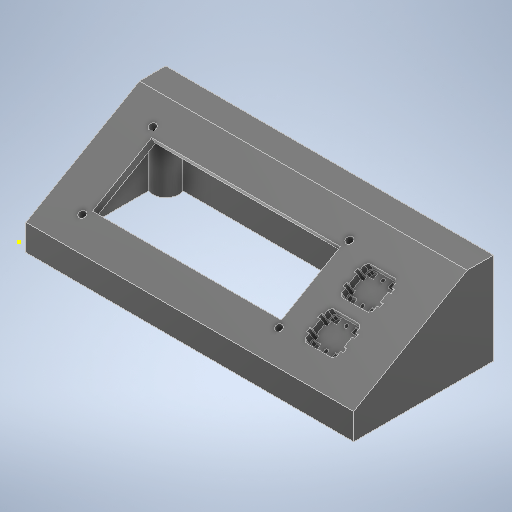
# Autodesk Inventor part: Control_Mount
Saved by Autodesk Inventor 2025.1 (Build 291241020, 241B)
## iProperties
Created: 2024-11-21
Part Number: Control_Mount
Material: PC/ABS Plastic
Document SubType Name: Modeling
Designer: leon-
Density: 1.1 g/cm^3
Appearance: Smooth - Black
Author: leon-
## iProperties of the stored document Control_Mount_3DPrint.ipt
Created: 2024-11-21
Part Number: Control_Mount_3DPrint
Material: Generic
Document SubType Name: Modeling
Designer: leon-
Density: 1 g/cm^3
Appearance: Default
Author: leon-
Autodesk Inventor part; units mm, degrees
ref_plane "YZ Plane" through (0, 0, 0) normal (1, 0, 0) x (0, 1, 0)
ref_plane "XZ Plane" through (0, 0, 0) normal (0, 1, 0) x (-1, 0, 0)
ref_plane "XY Plane" through (0, 0, 0) normal (0, 0, 1) x (1, 0, 0)
sketch "Sketch1" plane through (0, 0, 0) normal (1, 0, 0) x (0, 1, 0)
  line L0 (0, 0) -> (0, -53.3013)
  line L1 (0, -53.3013) -> (35, -53.3013)
  line L2 (35, -53.3013) -> (35, -43.3013)
  line L3 (35, -43.3013) -> (10, 0)
  line L4 (10, 0) -> (0, 0)
  point P0 (5, 0)
  dimension "d0" = 10
  dimension "d2" = 30
  dimension "d3" = 10
  dimension "d7" = 50
  constraints: 10 end point, 2 perpendicular, 1 midpoint, 1 parallel, 1 vertical
  measures "d0" distance of L1.end L2.end
  measures "d2" angle of L0 L3
  measures "d3" distance of L3.end L0.start
  measures "d7" distance of L2.end L3.end
extrude "Extrusion1" add sketch "Sketch1" along normal blind 125
shell "Shell1" thickness 3 removed faces 1 at (41.6667, 0, -17.7671)
sketch "Sketch2" plane through (0, 10, 0) normal (0, 0.8660254, 0.5) x (1, 0, 0)
  line L0 (15, 38) -> (87, 38)
  line L1 (87, 38) -> (87, 12)
  line L2 (87, 12) -> (15, 12)
  line L3 (15, 12) -> (15, 38)
  line L4 (125, 50) -> (125, 0) projected
  line L5 (0, 0) -> (125, 0) projected
  line L6 (0, 50) -> (0, 0) projected
  point P0 (0, -5)
  dimension "d8" = 26
  dimension "d9" = 72
  dimension "d11" = 12
  dimension "d25" = 15
  constraints: 8 end point, 2 parallel, 1 horizontal, 1 perpendicular
  measures "d8" distance of L0.end L1.end
  measures "d9" distance of L0.start L0.end
  measures "d11" distance between parallel lines of L5 L2
  measures "d25" distance between parallel lines of L6 L3
extrude "Extrusion2" cut sketch "Sketch2" against normal up to surface (3 mm away)
ref_plane "Work Plane1" through (87, 22.5, -21.6506) normal (0, 0.5, -0.8660254) x (-1, 0, 0)
ref_plane "Work Plane2" through (51, 16, -10.3923) normal (1, 0, 0) x (0, 0.5, -0.8660254)
sketch "Sketch3" plane through (0, 10, 0) normal (0, 0.8660254, 0.5) x (1, 0, 0)
  line L0 (51, 72.1423) -> (51, -22.2321) projected
  line L1 (-25, 25) -> (150, 25) projected
  point P0 (0, -5)
  point P1 (13, 40.8)
  point P2 (88, 40.8)
  point P3 (88, 9.8)
  point P4 (13, 9.8)
  dimension "d14" = 75
  dimension "d15" = 31
  dimension "d16" = 37
  dimension "d17" = 15.8
  constraints: 2 horizontal alignment, 2 vertical alignment
  measures "d14" distance of point (88, 40.8) point (13, 40.8)
  measures "d15" distance of point (88, 40.8) point (88, 9.8)
  measures "d16" distance from line of point (88, 40.8) L0
  measures "d17" distance from line of L1 point (88, 40.8)
hole "Hole1" at (13, 30.4, -35.3338) at (88, 30.4, -35.3338) at (88, 14.9, -8.487) at (13, 14.9, -8.487) direction (0, -0.8660254, -0.5) diameter 2.6 depth 3
sketch "Sketch4" plane through (3, 32, -44.1051) normal (0, -0.8660254, -0.5) x (1, 0, 0)
  line L0 (110, 7.1962) -> (90, 7.1962)
  line L1 (90, 7.1962) -> (90, 43.1962)
  line L2 (90, 43.1962) -> (110, 43.1962)
  line L3 (110, 43.1962) -> (110, 7.1962)
  line L4 (84, 37.1962) -> (12, 37.1962) projected
  line L5 (84, 11.1962) -> (84, 37.1962) projected
  line L6 (12, 11.1962) -> (84, 11.1962) projected
  point P0 (-3, 54.1962)
  dimension "d76" = 20
  dimension "d78" = 6
  dimension "d79" = 6
  dimension "d80" = 4
  constraints: 8 end point, 2 parallel, 1 horizontal, 1 perpendicular
  measures "d76" distance of L0.start L0.end
  measures "d78" distance between parallel lines of L4 L2
  measures "d79" distance between parallel lines of L5 L1
  measures "d80" distance between parallel lines of L6 L0
extrude "Extrusion3" add sketch "Sketch4" along normal blind 3
sketch "Sketch5" plane through (0, 10, 0) normal (0, 0.8660254, 0.5) x (1, 0, 0)
  line L0 (108, 22) -> (98, 22)
  line L1 (97, 21) -> (98, 22)
  line L2 (97, 21) -> (97, 11)
  line L3 (98, 10) -> (97, 11)
  line L4 (98, 10) -> (108, 10)
  line L5 (109, 11) -> (108, 10)
  line L6 (109, 11) -> (109, 21)
  line L7 (108, 22) -> (109, 21)
  circle A0 centre (103, 16) radius 3.5
  line L8 (87, 38) -> (87, 12) projected
  line L9 (87, 12) -> (15, 12) projected
  point P0 (0, -5)
  point P1 (98, 19.4445)
  point P2 (97, 16)
  dimension "d32" = 12
  dimension "d33" = 12
  dimension "d34" = 7
  dimension "d35" = 6
  dimension "d36" = 6
  dimension "d37" = 1
  dimension "d38" = 1
  dimension "d60" = 10
  dimension "d81" = 2
  constraints: 16 end point, 3 perpendicular, 2 horizontal alignment, 2 vertical alignment, 1 centre point, 1 midpoint
  measures "d32" distance between parallel lines of L6 L2
  measures "d33" distance between parallel lines of L4 L0
  measures "d34" diameter of A0
  measures "d35" distance from line of L6 A0.centre
  measures "d36" distance from line of L0 A0.centre
  measures "d37" horizontal distance of L0.start L6.end
  measures "d38" horizontal distance of L0.start L6.end
  measures "d60" distance from line of L8 point (97, 16)
  measures "d81" distance between parallel lines of L9 L4
ref_plane "Work Plane3" through (98, 19.7222, -16.8394) normal (1, 0, 0) x (0, 0, -1)
ref_plane "Work Plane4" through (92, 18.6328, -20.9325) normal (0, -0.8660254, -0.5) x (1, 0, 0)
extrude "Extrusion4" cut sketch "Sketch5" against normal up to surface (2.99 mm away) contours L7 L6 L5 L4 L3 L2 L1 L0 | A0
sketch "Sketch8" plane through (93, 20.1328, -23.5306) normal (0, 0.8660254, 0.5) x (1, 0, 0)
  line L0 (15.5, -5.9445) -> (12.8, -5.9445)
  line L1 (12.8, -5.9445) -> (12.8, -3.9445)
  line L2 (15.5, -4.6516) -> (15.5, -5.9445)
  line L3 (14.7929, -3.9445) -> (15.5, -4.6516)
  line L4 (12.8, -3.9445) -> (14.7929, -3.9445)
  circle A0 centre (10, -4.9445) radius 0.725
  line L5 (15.5, -14.2374) -> (14.7929, -14.9445)
  line L6 (15.5, -12.9445) -> (15.5, -14.2374)
  line L7 (16, -4.4445) -> (15, -3.4445)
  line L8 (16, -14.4445) -> (16, -4.4445)
  line L9 (15, -15.4445) -> (16, -14.4445)
  line L10 (5, -15.4445) -> (15, -15.4445)
  line L11 (4, -14.4445) -> (5, -15.4445)
  line L12 (4, -4.4445) -> (4, -14.4445)
  line L13 (5, -3.4445) -> (4, -4.4445)
  line L14 (15, -3.4445) -> (5, -3.4445)
  line L15 (5.2071, -3.9445) -> (7.2, -3.9445)
  line L16 (4.5, -4.6516) -> (5.2071, -3.9445)
  line L17 (4.5, -5.9445) -> (4.5, -4.6516)
  line L18 (7.2, -5.9445) -> (4.5, -5.9445)
  line L19 (7.2, -3.9445) -> (7.2, -5.9445)
  line L20 (4.5, -12.9445) -> (7.2, -12.9445)
  line L21 (4.5, -14.2374) -> (4.5, -12.9445)
  line L22 (5.2071, -14.9445) -> (4.5, -14.2374)
  line L23 (7.2, -14.9445) -> (5.2071, -14.9445)
  line L24 (7.2, -12.9445) -> (7.2, -14.9445)
  circle A1 centre (10, -13.9445) radius 0.725
  line L25 (12.8, -14.9445) -> (12.8, -12.9445)
  line L26 (14.7929, -14.9445) -> (12.8, -14.9445)
  line L27 (15.5, -14.2374) -> (14.7929, -14.9445)
  line L28 (15.5, -12.9445) -> (15.5, -14.2374)
  line L29 (12.8, -12.9445) -> (15.5, -12.9445)
  line L30 (15.5, -4.6516) -> (15.5, -5.9445)
  line L31 (14.7929, -3.9445) -> (15.5, -4.6516)
  line L32 (12.8, -3.9445) -> (14.7929, -3.9445)
  line L33 (12.8, -5.9445) -> (12.8, -3.9445)
  line L34 (15.5, -5.9445) -> (12.8, -5.9445)
  circle A2 centre (10, -9.4445) radius 3.5
  line L35 (-6, 12.5555) -> (-6, -13.4445) projected
  line L36 (-6, -13.4445) -> (-78, -13.4445) projected
  point P0 (-93, -30.4445)
  point P1 (7.2, -4.9445)
  point P2 (7.2, -13.9445)
  point P3 (12.8, -13.9445)
  point P4 (12.8, -4.9445)
  point P5 (12.8, -4.9445)
  point P6 (4, -9.4445)
  point P7 (4.5, -13.5909)
  dimension "d39" = 7
  dimension "d40" = 1.45
  dimension "d41" = 1.45
  dimension "d42" = 4.5
  dimension "d43" = 4.5
  dimension "d44" = 2.7
  dimension "d45" = 2
  dimension "d46" = 0.5
  dimension "d47" = 135
  dimension "d48" = 1.9929
  dimension "d49" = 0.5
  dimension "d50" = 10
  dimension "d51" = 10
  dimension "d52" = 6
  dimension "d53" = 135
  dimension "d54" = 1
  dimension "d55" = 0.5
  dimension "d56" = 1
  dimension "d57" = 12
  dimension "d58" = 0.5
  dimension "d59" = 6
  dimension "d62" = 10
  dimension "d82" = 2
  constraints: 70 end point, 15 equal length, 9 vertical, 7 midpoint, 6 vertical alignment, 5 horizontal, 4 horizontal alignment, 3 centre point
  measures "d39" diameter of A2
  measures "d40" diameter of A1
  measures "d41" diameter of A0
  measures "d42" distance of A2.centre A0.centre
  measures "d43" distance of A2.centre A1.centre
  measures "d44" distance of L19.end L18.end
  measures "d45" distance of L19.start L19.end
  measures "d46" distance between parallel lines of L14 L15
  measures "d47" angle of L17 L16
  measures "d48" distance of L15.start L19.start
  measures "d49" distance between parallel lines of L10 L23
  measures "d50" distance of L7.end L14.end
  measures "d51" distance of L9.end L7.start
  measures "d52" distance from line of A2.centre L8
  measures "d53" angle of L8 L7
  measures "d54" horizontal distance of L7.end L7.start
  measures "d55" distance between parallel lines of L12 L17
  measures "d56" distance from line of L14.end L12
  measures "d57" distance between parallel lines of L10 L14
  measures "d58" distance between parallel lines of L8 L28
  measures "d59" distance from line of L14 A2.centre
  measures "d62" distance between parallel lines of L35 L12
  measures "d82" distance between parallel lines of L10 L36
extrude "Extrusion5" cut sketch "Sketch8" against normal blind 2 contours L0 L1 L4 L3 L2 | A0 | L5 L26 L25 L29 L6 | L15 L19 L18 L17 L16 | L20 L24 L23 L22 L21 | A1
sketch "Sketch9" plane through (98, 18.4106, -20.5476) normal (0, 0.8660254, 0.5) x (1, 0, 0)
  point P0 (-98, -27)
sketch "Sketch10" plane through (98, 18.4106, -20.5476) normal (0, 0.8660254, 0.5) x (1, 0, 0)
  point P0 (-98, -27)
sketch "Sketch11" plane through (98, 18.4106, -20.5476) normal (0, 0.8660254, 0.5) x (1, 0, 0)
  line L0 (-2, -2.75) -> (0, -2.75)
  line L1 (0, -2.75) -> (0, -4.25)
  line L2 (0, -4.25) -> (-2, -4.25)
  line L3 (-2, -4.25) -> (-2, -2.75)
  line L4 (-1, -11) -> (-1, -1) projected
  line L5 (0, 0) -> (10, 0) projected
  line L6 (-2, -7.75) -> (0, -7.75)
  line L7 (0, -7.75) -> (0, -9.25)
  line L8 (0, -9.25) -> (-2, -9.25)
  line L9 (-2, -9.25) -> (-2, -7.75)
  line L10 (10, -2.75) -> (12, -2.75)
  line L11 (12, -2.75) -> (12, -4.25)
  line L12 (12, -4.25) -> (10, -4.25)
  line L13 (10, -4.25) -> (10, -2.75)
  line L14 (10, -7.75) -> (12, -7.75)
  line L15 (12, -7.75) -> (12, -9.25)
  line L16 (12, -9.25) -> (10, -9.25)
  line L17 (10, -9.25) -> (10, -7.75)
  line L18 (10, -12) -> (0, -12) projected
  line L19 (11, -1) -> (11, -11) projected
  point P0 (-98, -27)
  point P1 (-2, -3.5)
  point P2 (-2, -8.5)
  point P3 (12, -3.5)
  point P4 (12, -8.5)
  point P5 (0, -3.5)
  point P6 (0, -8.5)
  point P7 (10, -3.5)
  point P8 (10, -8.5)
  dimension "d64" = 1
  dimension "d65" = 1.5
  dimension "d66" = 2.75
  dimension "d67" = 1
  dimension "d68" = 1.5
  dimension "d69" = 2.75
  dimension "d70" = 1
  dimension "d71" = 1
  constraints: 32 end point, 8 midpoint, 8 parallel, 4 horizontal, 4 horizontal alignment, 4 perpendicular, 4 vertical alignment, 1 point on line
  measures "d64" distance between parallel lines of L4 L3
  measures "d65" distance between parallel lines of L2 L0
  measures "d66" distance between parallel lines of L5 L0
  measures "d67" distance between parallel lines of L4 L1
  measures "d68" distance between parallel lines of L8 L6
  measures "d69" distance between parallel lines of L18 L8
  measures "d70" distance between parallel lines of L19 L13
  measures "d71" distance between parallel lines of L19 L11
extrude "Extrusion6" cut sketch "Sketch11" along normal blind 10 and the other way blind 10
ref_plane "Work Plane5" through (113, 19.4019, -22.2846) normal (0, 0.5, -0.8660254) x (-1, 0, 0)
mirror "Mirror1" about plane through (113, 19.4019, -22.2846) normal (0, 0.5, -0.8660254) of "Extrusion4", "Extrusion5", "Extrusion6"
sketch "Sketch12" plane through (0, 0, -53.3013) normal (0, -1, 0) x (1, 0, 0)
  circle A0 centre (120, 5) radius 5
  line L0 (125, 53.3013) -> (125, 0) projected
  line L1 (0, 0) -> (125, 0) projected
  point P0 (0, 53.3013)
  dimension "d83" = 10
  dimension "d84" = 5
  dimension "d85" = 5
  constraints: 1 centre point
  measures "d83" diameter of A0
  measures "d84" distance from line of L0 A0.centre
  measures "d85" distance from line of L1 A0.centre
extrude "Extrusion7" add sketch "Sketch12" against normal up to surface (32 mm away) contours A0
sketch "Sketch13" plane through (0, 0, -53.3013) normal (0, -1, 0) x (1, 0, 0)
  circle A0 centre (120, 48.3013) radius 5
  line L0 (0, 53.3013) -> (125, 53.3013) projected
  line L1 (125, 53.3013) -> (125, 0) projected
  dimension "d88" = 10
  dimension "d89" = 5
  dimension "d90" = 5
  constraints: 1 centre point
  measures "d88" diameter of A0
  measures "d89" distance from line of L0 A0.centre
  measures "d90" distance from line of L1 A0.centre
extrude "Extrusion8" add sketch "Sketch13" against normal up to surface contours A0 surface through (0, 32.4019, -44.8013) normal (0, 0.8660254, 0.5)
sketch "Sketch14" plane through (0, 0, -53.3013) normal (0, -1, 0) x (1, 0, 0)
  arc A0 (122, 9.5826) -> (115.4174, 3) centre (120, 5) ccw projected
  arc A1 (115.4174, 50.3013) -> (122, 43.7187) centre (120, 48.3013) ccw projected
  point P0 (0, 53.3013)
  constraints: 2 coincident
hole "Hole2" at (120, 0, -48.3013) at (120, 0, -5) direction (0, 1, 0) diameter 4.3 depth 8
ref_plane "Work Plane6" through (62.5, 0, 0) normal (1, 0, 0) x (0, 0, -1)
mirror "Mirror2" about plane through (62.5, 0, 0) normal (1, 0, 0) of "Extrusion8", "Extrusion7", "Hole2"
body "Solid1"
